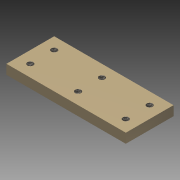
# Autodesk Inventor part: 13_0204_063
Saved by Autodesk Inventor 2012 SP1 (Build 160190100, 190)
## iProperties
Created: 2013-04-30
Part Number: 13_0204_063
Material: Default
Document SubType Name: Modeling
Designer: vogel
Density: 1 g/cm^3
Author: vogel
Autodesk Inventor part; units mm, degrees
ref_plane "YZ Plane" through (0, 0, 0) normal (1, 0, 0) x (0, 1, 0)
ref_plane "XZ Plane" through (0, 0, 0) normal (0, 1, 0) x (-1, 0, 0)
ref_plane "XY Plane" through (0, 0, 0) normal (0, 0, 1) x (1, 0, 0)
sketch "Skizze1" plane through (0, 0, 0) normal (0, 0, 1) x (1, 0, 0)
  line L0 (0, 0) -> (50, 0)
  line L1 (50, 0) -> (50, 20)
  line L2 (50, 20) -> (0, 20)
  line L3 (0, 20) -> (0, 0)
  dimension "d0" = 20
  dimension "d1" = 50
  constraints: 8 end point, 2 parallel, 1 horizontal, 1 perpendicular
  measures "d0" distance of L2.end L0.start
  measures "d1" distance of L0.start L0.end
extrude "Extrusion1" add sketch "Skizze1" along normal blind 4
sketch "Skizze2" plane through (0, 0, 4) normal (0, 0, 1) x (1, 0, 0)
  line L0 (0, 0) -> (0, 20) projected
  line L1 (50, 0) -> (0, 0) projected
  line L2 (0, 20) -> (50, 20) projected
  line L3 (5, 15) -> (45, 15)
  line L4 (45, 15) -> (45, 5)
  line L5 (45, 5) -> (5, 5)
  line L6 (5, 5) -> (5, 15)
  line L7 (25, 0) -> (25, 20)
  line L8 (0, 10) -> (6.0209, 10)
  point P0 (25, 5)
  point P1 (25, 15)
  dimension "d4" = 10
  dimension "d5" = 5
  constraints: 12 end point, 5 midpoint, 4 coincident, 2 parallel, 2 perpendicular, 2 point on line, 1 horizontal, 2 other
  measures "d4" distance of L5.end L3.start
  measures "d5" distance between parallel lines of L0 L6
hole "Bohrung1" at (5, 15, 4) at (5, 5, 4) at (25, 5, 4) at (25, 15, 4) at (45, 15, 4) at (45, 5, 4) direction (0, 0, -1) diameter 2.459 end through all thread size "M3x0.5" class "6H" standard "ISO Metric profile"
